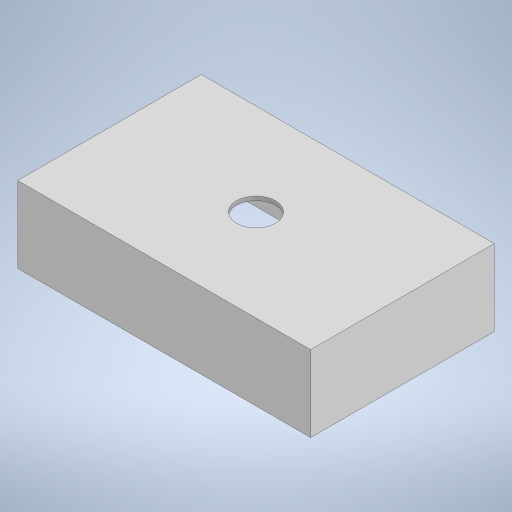
# Autodesk Inventor part: top batt cage
Saved by Autodesk Inventor 2024 (Build 280153000, 153)
## iProperties
Created: 2025-05-11
Part Number: top batt cage
Material: Generic
Document SubType Name: Modeling
Designer: arikm
Density: 1 g/cm^3
Appearance: Default
Author: arikm
Autodesk Inventor part; units mm, degrees
ref_plane "YZ Plane" through (0, 0, 0) normal (1, 0, 0) x (0, 1, 0)
ref_plane "XZ Plane" through (0, 0, 0) normal (0, 1, 0) x (-1, 0, 0)
ref_plane "XY Plane" through (0, 0, 0) normal (0, 0, 1) x (1, 0, 0)
sketch "Sketch1" plane through (0, 0, 0) normal (0, 1, 0) x (-1, 0, 0)
  line L0 (0, 0) -> (69, 0)
  line L1 (69, 0) -> (69, -41)
  line L2 (69, -41) -> (0, -41)
  line L3 (0, -41) -> (0, 0)
  line L4 (-3, 3) -> (72, 3)
  line L5 (72, 3) -> (72, -44)
  line L6 (72, -44) -> (-3, -44)
  line L7 (-3, -44) -> (-3, 3)
  dimension "d0" = 69
  dimension "d1" = 41
  dimension "d2" = 3
  constraints: 16 end point, 4 parallel, 2 perpendicular, 1 horizontal, 3 other
  measures "d0" distance of L1.end L2.end
  measures "d1" distance of L0.end L1.end
  measures "d2" distance between parallel lines of L3 L7
extrude "Extrusion1" add sketch "Sketch1" along normal blind 18.5
sketch "Sketch2" plane through (0, 18.5, 0) normal (0, 1, 0) x (1, 0, 0)
  line L0 (0, 0) -> (-69, 0) projected
  line L1 (-69, 41) -> (0, 41) projected
  line L2 (-69, 0) -> (0, 0)
  line L3 (0, 0) -> (0, 41)
  line L4 (0, 41) -> (-69, 41)
  line L5 (-69, 41) -> (-69, 0)
  line L6 (0.2, 41.2) -> (0.2, -0.2)
  line L7 (0.2, -0.2) -> (-69.2, -0.2)
  line L8 (-69.2, -0.2) -> (-69.2, 41.2)
  line L9 (-69.2, 41.2) -> (0.2, 41.2)
  dimension "d5" = 0.2
  constraints: 16 end point, 4 parallel, 2 perpendicular, 1 horizontal, 3 other
  measures "d5" distance between parallel lines of L3 L6
extrude "Extrusion2" cut sketch "Sketch2" against normal blind 18.5
sketch "Sketch3" plane through (0, 18.5, 0) normal (0, 1, 0) x (1, 0, 0)
  line L0 (-72, -3) -> (3, -3) projected
  line L1 (3, -3) -> (3, 44) projected
  line L2 (-72, -3) -> (3, -3)
  line L3 (3, -3) -> (3, 44)
  line L4 (3, 44) -> (-72, 44)
  line L5 (-72, 44) -> (-72, -3)
  point P0 (0, 0)
  constraints: 8 end point, 2 parallel, 1 horizontal, 1 perpendicular
extrude "Extrusion3" add sketch "Sketch3" along normal blind 1
sketch "Sketch4" plane through (0, 19.5, 0) normal (0, 1, 0) x (1, 0, 0)
  line L0 (3, -3) -> (3, 44) projected
  line L1 (3, 44) -> (-72, 44) projected
  line L2 (3, -3) -> (-72, 44)
  circle A0 centre (-34.5, 20.5) radius 5
  point P0 (0, 0)
  dimension "d10" = 10
  constraints: 2 end point, 1 centre point, 1 midpoint
  measures "d10" diameter of A0
extrude "Extrusion4" cut sketch "Sketch4" against normal blind 1 contours A0 L2 | L2 A0
body "Solid1"
